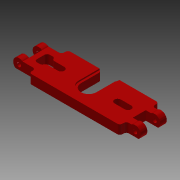
# Autodesk Inventor part: 6mm_groove_mounting_plate
Saved by Autodesk Inventor 2014 (Build 180170000, 170)
## iProperties
Created: 2016-10-19
Part Number: 6mm_groove_mounting_plate
Material: Generic
Document SubType Name: Modeling
Designer: Rubén
Density: 1 g/cm^3
Appearance: Smooth - Red
Author: Rubén
Autodesk Inventor part; units mm, degrees
ref_plane "YZ Plane" through (0, 0, 0) normal (1, 0, 0) x (0, 1, 0)
sketch "Sketch1" plane through (0, 0, 0) normal (0, 1, 0) x (-1, 0, 0)
  line L0 (68, 30) -> (2, 30)
  line L1 (0, 28) -> (0, 2)
  line L2 (32, 0) -> (32, 16)
  line L3 (38, 22) -> (38, 22)
  line L4 (44, 16) -> (44, 0)
  line L5 (2, 0) -> (32, 0)
  line L6 (44, 0) -> (68, 0)
  line L7 (8.7, 17.5) -> (16.7, 17.5)
  line L8 (19.2, 15) -> (19.2, 15)
  line L9 (16.7, 12.5) -> (8.7, 12.5)
  line L10 (6.2, 15) -> (6.2, 15)
  line L11 (68, 17.5) -> (60.2, 17.5)
  line L12 (57.7, 15) -> (57.7, 15)
  line L13 (60.2, 12.5) -> (68, 12.5)
  line L14 (70, 2) -> (70, 10.5)
  line L15 (70, 19.5) -> (70, 28)
  line L16 (70, 17.5) -> (70, 12.5) construction
  line L17 (19.2, 17.5) -> (57.7, 17.5) construction
  line L18 (57.7, 12.5) -> (19.2, 12.5) construction
  line L19 (32, 0) -> (44, 0) construction
  arc A0 (2, 30) -> (0, 28) centre (2, 28) ccw
  arc A1 (0, 2) -> (2, 0) centre (2, 2) ccw
  arc A2 (68, 0) -> (70, 2) centre (68, 2) ccw
  arc A3 (70, 28) -> (68, 30) centre (68, 28) ccw
  arc A4 (68, 17.5) -> (70, 19.5) centre (68, 19.5) ccw
  arc A5 (70, 10.5) -> (68, 12.5) centre (68, 10.5) ccw
  arc A6 (8.7, 17.5) -> (6.2, 15) centre (8.7, 15) ccw
  arc A7 (6.2, 15) -> (8.7, 12.5) centre (8.7, 15) ccw
  arc A8 (16.7, 12.5) -> (19.2, 15) centre (16.7, 15) ccw
  arc A9 (19.2, 15) -> (16.7, 17.5) centre (16.7, 15) ccw
  arc A10 (60.2, 17.5) -> (57.7, 15) centre (60.2, 15) ccw
  arc A11 (57.7, 15) -> (60.2, 12.5) centre (60.2, 15) ccw
  arc A12 (38, 22) -> (32, 16) centre (38, 16) ccw
  arc A13 (44, 16) -> (38, 22) centre (38, 16) ccw
  point P0 (0, 0)
  point P1 (70, 30)
  point P2 (0, 30)
  point P3 (32, 22)
  point P4 (6.2, 17.5)
  dimension "d0" = 12
  dimension "d1" = 70
  dimension "d2" = 5
  dimension "d3" = 32
  dimension "d4" = 13
  dimension "d5" = 6.2
  dimension "d6" = 12.3
  dimension "d7" = 30
  dimension "d8" = 22
  dimension "d9" = 2
  dimension "d10" = 2.5
  dimension "d11" = 6
  constraints: 40 end point, 28 point on circle, 28 tangent, 22 point on line, 14 centre point, 12 perpendicular, 11 equal radius, 7 parallel, 6 horizontal, 2 collinear
  measures "d0" distance between parallel lines of L4 L2
  measures "d1" distance of point (70, 30) point (0, 30)
  measures "d2" distance of L17.end L18.start
  measures "d3" distance of point (0, 0) L2.start
  measures "d4" distance of point (6.2, 17.5) L17.start
  measures "d5" distance between parallel lines of L10 L1
  measures "d6" distance of L16.start L17.end
  measures "d7" distance of point (0, 30) point (0, 0)
  measures "d8" distance of L2.start point (32, 22)
  measures "d9" radius of A0
  measures "d10" radius of A6
  measures "d11" radius of A12
extrude "Extrusion1" add sketch "Sketch1" along normal blind 7
sketch "Sketch2" plane through (0, 7, 0) normal (0, 1, 0) x (1, 0, 0)
  line L0 (-32, 0) -> (-32, -16) projected
  arc A0 (-44, -16) -> (-32, -16) centre (-38, -16) ccw projected
  line L1 (-44, -16) -> (-44, 0) projected
  line L2 (-44, 0) -> (-68, 0) projected
  arc A1 (-68, 0) -> (-70, -2) centre (-68, -2) ccw projected
  line L3 (-70, -2) -> (-70, -10.5) projected
  arc A2 (-70, -10.5) -> (-68, -12.5) centre (-68, -10.5) ccw projected
  line L4 (-68, -12.5) -> (-60.2, -12.5) projected
  arc A3 (-60.2, -17.5) -> (-60.2, -12.5) centre (-60.2, -15) ccw projected
  line L5 (-60.2, -17.5) -> (-68, -17.5) projected
  arc A4 (-68, -17.5) -> (-70, -19.5) centre (-68, -19.5) ccw projected
  line L6 (-70, -19.5) -> (-70, -28) projected
  arc A5 (-70, -28) -> (-68, -30) centre (-68, -28) ccw projected
  line L7 (-68, -30) -> (-2, -30) projected
  arc A6 (-2, -30) -> (0, -28) centre (-2, -28) ccw projected
  line L8 (0, -28) -> (0, -2) projected
  arc A7 (0, -2) -> (-2, 0) centre (-2, -2) ccw projected
  line L9 (-2, 0) -> (-32, 0) projected
  line L10 (-45.6, -1.6) -> (-45.6, -16)
  arc A8 (-45.6, -16) -> (-30.4, -16) centre (-38, -16) ccw
  line L11 (-30.4, -16) -> (-30.4, -1.6)
  line L12 (-30.4, -1.6) -> (-2, -1.6)
  arc A9 (-1.6, -2) -> (-2, -1.6) centre (-2, -2) ccw
  line L13 (-1.6, -2) -> (-1.6, -28)
  arc A10 (-2, -28.4) -> (-1.6, -28) centre (-2, -28) ccw
  line L14 (-2, -28.4) -> (-68, -28.4)
  arc A11 (-68.4, -28) -> (-68, -28.4) centre (-68, -28) ccw
  line L15 (-68.4, -28) -> (-68.4, -19.5)
  arc A12 (-68, -19.1) -> (-68.4, -19.5) centre (-68, -19.5) ccw
  line L16 (-68, -19.1) -> (-60.2, -19.1)
  arc A13 (-60.2, -19.1) -> (-60.2, -10.9) centre (-60.2, -15) ccw
  line L17 (-60.2, -10.9) -> (-68, -10.9)
  arc A14 (-68.4, -10.5) -> (-68, -10.9) centre (-68, -10.5) ccw
  line L18 (-68.4, -10.5) -> (-68.4, -2)
  arc A15 (-68, -1.6) -> (-68.4, -2) centre (-68, -2) ccw
  line L19 (-68, -1.6) -> (-45.6, -1.6)
  line L20 (-45.6, -1.6) -> (-45.6, 0)
  line L21 (-30.4, -1.6) -> (-30.4, 0)
  point P0 (0, 0)
  dimension "d14" = 1.6
  constraints: 24 end point, 16 point on circle, 8 centre point, 2 point on line, 1 parallel, 1 perpendicular, 17 other
  measures "d14" distance between parallel lines of L1 L10
extrude "Extrusion2" cut sketch "Sketch2" against normal blind 1 contours L9 L21 L11 A8 L10 L20 L2 L1 A0 L0
fillet "Fillet1" radius 2 2 edges at (-32, 3, 0) (-44, 3, 0)
sketch "Sketch3" plane through (-2, 0, 0) normal (0, 0, -1) x (-1, 0, 0)
  line L0 (-2, 0) -> (-2, 7) projected
  line L1 (-2, 7) -> (-6, 7)
  line L2 (-6, 7) -> (-6, 0)
  line L3 (-6, 0) -> (-2, 0)
  line L4 (-6, 3.5) -> (-13.2011, 3.5) construction
  arc A0 (-6, 7) -> (-11.5, 0) centre (-8.75, 3.5) ccw
  circle A1 centre (-8.75, 3.5) radius 1.6
  circle A2 centre (-8.75, 3.5) radius 2.75 construction
  line L5 (-11.5, 0) -> (-6, 0)
  arc A3 (-11.5, 0) -> (-6, 0) centre (-8.75, 3.5) ccw construction
  dimension "d18" = 4
  dimension "d19" = 5.5
  dimension "d20" = 3.2
  constraints: 10 end point, 6 point on circle, 4 centre point, 3 parallel, 2 coincident, 2 perpendicular, 1 midpoint, 1 tangent
  measures "d18" distance of L0.end L1.end
  measures "d19" diameter of A2
  measures "d20" diameter of A1
ref_plane "Work Plane3" through (-57.7, 7, 5) normal (0, 0, 1) x (1, 0, 0)
ref_plane "Work Plane2" through (-57.7, 7, 10) normal (0, 0, 1) x (1, 0, 0)
extrude "Extrusion3" add sketch "Sketch3" against normal up to surface (5 mm away) from surface at -5
mirror "Mirror1" about plane through (-57.7, 7, 15) normal (0, 0, 1) of "Extrusion3"
ref_plane "Work Plane4" through (-38, 6, 22) normal (1, 0, 0) x (0, 1, 0)
mirror "Mirror2" about plane through (-38, 6, 22) normal (1, 0, 0) of "Extrusion3", "Mirror1"
sketch "Sketch4" plane through (0, 7, 0) normal (0, 1, 0) x (1, 0, 0)
  line L0 (-70, -2) -> (-70, -10.5) projected
  line L1 (-70, -19.5) -> (-70, -28) projected
  line L2 (-76, -10) -> (-80, -10) projected
  line L3 (-76, -5) -> (-76, -10) projected
  line L4 (-76, -5) -> (-80, -5) projected
  line L5 (-80, -5) -> (-80, -10) projected
  line L6 (-76, -20) -> (-80, -20) projected
  line L7 (-80, -25) -> (-80, -20) projected
  line L8 (-76, -25) -> (-80, -25) projected
  line L9 (-76, -25) -> (-76, -20) projected
  line L10 (-76, -5) -> (-70, -5)
  line L11 (-76, -10) -> (-70, -10)
  line L12 (-76, -20) -> (-70, -20)
  line L13 (-76, -25) -> (-70, -25)
  line L14 (-80, -20) -> (-80, -10)
  line L15 (-76, -10) -> (-76, -20)
  point P0 (0, 0)
  constraints: 12 end point, 5 perpendicular, 4 point on line, 1 collinear
extrude "Extrusion4" add sketch "Sketch4" against normal up to surface (7 mm away) contours L0 L11 L3 L10 | L15 L6 L14 L2 | L12 L1 L13 L9
fillet "Fillet2" radius 2 8 edges at (-70, 3.5, 20) (-76, 3.5, 20) (-76, 3.5, 10) (-70, 3.5, 10) (-70, 3.5, 5) (-70, 3.5, 25) (0, 3.5, 5) (0, 3.5, 25)
ref_plane "Work Plane1" through (-57.7, 7, 15) normal (0, 0, 1) x (1, 0, 0)
body "Solid1"
